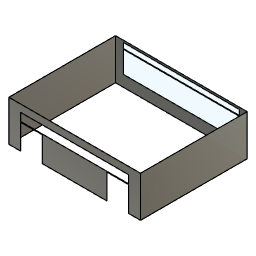
教室【窓とドアの大体のサイズだよー】※位置は教室で変わったりするので注意 (Autodesk Fusion 360 design; units mm, degrees)
Autodesk Fusion 360 part; units mm, degrees
sketch "スケッチ1" plane through (0, 0, 0) normal (0, 1, 0) x (1, 0, 0)
sketch "スケッチ2" plane through (0, 0, 0) normal (0, 0, 1) x (1, 0, 0)
  line L0 (0, 0) -> (-10000, 0)
  line L1 (-10000, 0) -> (-10000, 8100)
  line L2 (-10000, 8100) -> (0, 8100)
  line L3 (0, 8100) -> (0, 0)
  line L4 (10, -10) -> (-10010, -10)
  line L5 (-10010, -10) -> (-10010, 8110)
  line L6 (-10010, 8110) -> (10, 8110)
  line L7 (10, 8110) -> (10, -10)
  point P0 (10, -10)
  dimension "d1" = 10000
  dimension "d2" = 8100
  dimension "d4" = 10020
  dimension "d5" = 8120
  constraint horizontal L0
  constraint vertical L1
  constraint horizontal L2
  constraint vertical L3
  constraint coincident L0.start L3.end
  constraint horizontal L4
  constraint vertical L5
  constraint horizontal L6
  constraint vertical L7
  constraint coincident P0 L4.start
  measures "d1" distance of L0.start L0.end
  measures "d2" distance of L0.start L2.end
  measures "d4" distance of L5.end L6.end
  measures "d5" distance of L4.end L5.end
extrude "押し出し1" add sketch "スケッチ2" along normal blind 3100
sketch "スケッチ3" plane through (0, -10, 0) normal (0, -1, 0) x (1, 0, 0)
  line L0 (-10010, 0) -> (10, 0)
  line L1 (10, 0) -> (10, 3100)
  line L2 (10, 3100) -> (-10010, 3100)
  line L3 (-10010, 3100) -> (-10010, 0)
  line L4 (-900, 0) -> (-2550, 0)
  line L5 (-2550, 0) -> (-2550, 1900)
  line L6 (-2550, 1900) -> (-900, 1900)
  line L7 (-900, 1900) -> (-900, 0)
  line L8 (-9110, 0) -> (-7460, 0)
  line L9 (-7460, 0) -> (-7460, 1900)
  line L10 (-7460, 1900) -> (-9110, 1900)
  line L11 (-9110, 1900) -> (-9110, 0)
  line L12 (-900, 1950) -> (-9110, 1950)
  line L13 (-9110, 1950) -> (-9110, 2550)
  line L14 (-9110, 2550) -> (-900, 2550)
  line L15 (-900, 2550) -> (-900, 1950)
  point P0 (-900, 0)
  point P1 (-9110, 0)
  point P2 (-900, 1900)
  point P3 (-900, 1950)
  dimension "d8" = 900
  dimension "d9" = 900
  dimension "d12" = 1650
  dimension "d13" = 1900
  dimension "d14" = 50
  dimension "d15" = 600
  constraint coincident L0 P0
  constraint horizontal L4
  constraint vertical L5
  constraint horizontal L6
  constraint vertical L7
  constraint coincident P0 L4.start
  constraint coincident L0 P1
  constraint horizontal L8
  constraint vertical L9
  constraint horizontal L10
  constraint vertical L11
  constraint coincident P1 L8.start
  constraint coincident P2 L6.end
  constraint horizontal L12
  constraint vertical L13
  constraint horizontal L14
  constraint vertical L15
  constraint coincident P3 L12.start
  measures "d8" distance of origin L4.start
  measures "d9" distance of L0.start L8.start
  measures "d12" distance of P1 L8.end
  measures "d13" distance of L8.end L9.end
  measures "d14" distance of P2 P3
  measures "d15" distance of L12.end L13.end
extrude "押し出し2" cut sketch "スケッチ3" against normal blind 200 contours L0 L8 L9 L10 L11 | L0 L4 L5 L6 L7 | L12 L13 L14 L15
sketch "スケッチ4" plane through (0, 8110, 0) normal (0, 1, 0) x (-1, 0, 0)
  line L0 (-10, 0) -> (10010, 0)
  line L1 (10010, 0) -> (10010, 3100)
  line L2 (10010, 3100) -> (-10, 3100)
  line L3 (-10, 3100) -> (-10, 0)
sketch "スケッチ5" plane through (-5000, 8110, 1550) normal (0, 1, 0) x (-1, 0, 0)
  line L0 (-5010, 1550) -> (-5010, -1550)
  line L1 (-4410, 1400) -> (4400, 1400)
  line L2 (4400, 1400) -> (4400, 1000)
  line L3 (4400, 1000) -> (-4410, 1000)
  line L4 (-4410, 1000) -> (-4410, 1400)
  line L5 (-4410, 950) -> (4400, 950)
  line L6 (4400, 950) -> (4400, -700)
  line L7 (4400, -700) -> (-4410, -700)
  line L8 (-4410, -700) -> (-4410, 950)
  line L9 (-5010, -1550) -> (5010, -1550)
  point P0 (-4410, 1400)
  point P1 (-5010, 1550)
  point P2 (4410, 1400)
  point P3 (5010, 1550)
  point P4 (-4410, 950)
  dimension "d18" = 600
  dimension "d19" = 150
  dimension "d20" = 600
  dimension "d21" = 50
  dimension "d23" = 1650
  constraint horizontal L1
  constraint vertical L2
  constraint horizontal L3
  constraint vertical L4
  constraint coincident P0 L1.start
  constraint horizontal L5
  constraint vertical L6
  constraint horizontal L7
  constraint vertical L8
  constraint coincident P4 L5.start
  measures "d18" distance of P0 L0
  measures "d19" vertical distance of P0 L0.start
  measures "d20" horizontal distance of P2 P3
  measures "d21" distance of L3.end P4
  measures "d23" distance of P4 L7.end
extrude "押し出し3" cut sketch "スケッチ5" against normal blind 900
